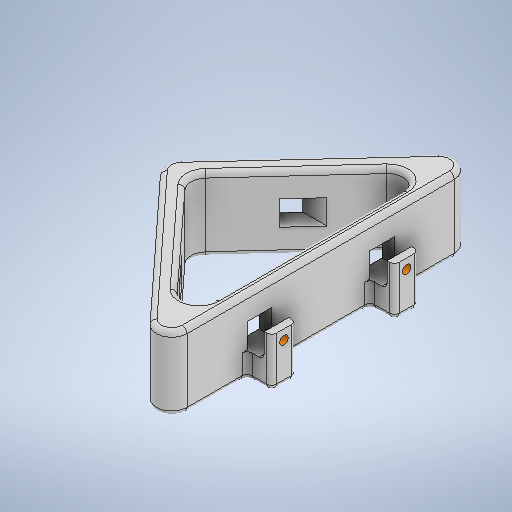
# Autodesk Inventor part: pare-chocs
Saved by Autodesk Inventor 2025 (Build 290162000, 162)
## iProperties
Created: 2024-10-10
Part Number: pare-chocs
Material: Générique
Document SubType Name: Modeling
Designer: chass
Density: 1 g/cm^3
Appearance: Par défaut
Author: chass
## iProperties of the stored document pare-chocs_Impression 3D.ipt
Created: 2025-01-09
Part Number: pare-chocs_Impression 3D
Material: Générique
Document SubType Name: Modeling
Designer: chass
Density: 1 g/cm^3
Appearance: Par défaut
Author: chass
Autodesk Inventor part; units mm, degrees
ref_plane "YZ Plane" through (0, 0, 0) normal (1, 0, 0) x (0, 1, 0)
ref_plane "XZ Plane" through (0, 0, 0) normal (0, 1, 0) x (-1, 0, 0)
ref_plane "XY Plane" through (0, 0, 0) normal (0, 0, 1) x (1, 0, 0)
sketch "Esquisse1" plane through (0, 0, 0) normal (1, 0, 0) x (0, 1, 0)
  line L0 (-2.5, 65) -> (2.5, 65)
  line L1 (2.5, 65) -> (2.5, -65)
  line L2 (2.5, -65) -> (-2.5, -65)
  line L3 (-2.5, -65) -> (-2.5, 65)
  line L4 (2.5, 65) -> (-2.5, -65)
  line L5 (2.5, -65) -> (-2.5, 65)
  point P0 (0, 0)
  point P1 (0, 0)
  point P2 (0, 0)
  dimension "d0" = 130
  dimension "d1" = 5
  constraints: 12 end point, 2 midpoint, 2 parallel, 1 coincident, 1 horizontal, 1 perpendicular
  measures "d0" distance of L0.end L1.end
  measures "d1" distance of L1.end L2.end
extrude "Extrusion1" add sketch "Esquisse1" along normal blind 5
sketch "Esquisse2" plane through (5, 0, 0) normal (1, 0, 0) x (0, 0, -1)
  line L0 (65, 2.5) -> (-65, 2.5) projected
  line L1 (-65, -2.5) -> (65, -2.5) projected
  line L2 (-30, 2.5) -> (-20, 2.5)
  line L3 (-20, 2.5) -> (-20, -2.5)
  line L4 (-20, -2.5) -> (-30, -2.5)
  line L5 (-30, -2.5) -> (-30, 2.5)
  line L6 (0, 13) -> (0, -16)
  line L7 (30, 2.5) -> (20, 2.5)
  line L8 (20, 2.5) -> (20, -2.5)
  line L9 (20, -2.5) -> (30, -2.5)
  line L10 (30, -2.5) -> (30, 2.5)
  point P0 (0, 0)
  point P1 (-20, 2.5)
  point P2 (30, -2.5)
  point P3 (30, 2.5)
  point P4 (20, 2.5)
  point P5 (20, -2.5)
  dimension "d4" = 10
  dimension "d5" = 20
  constraints: 18 end point, 4 symmetric about line, 3 point on line, 2 parallel, 1 horizontal, 1 perpendicular, 1 vertical
  measures "d4" distance between parallel lines of L3 L5
  measures "d5" distance between parallel lines of L3 L6
extrude "Extrusion2" add sketch "Esquisse2" along normal blind 10 contours L10 L1 L8 L0 | L3 L1 L5 L0
sketch "Esquisse3" plane through (0, 2.5, 65) normal (0, 1, 0) x (1, 0, 0)
  line L0 (15, 45) -> (15, 35) projected
  line L1 (5, 45) -> (15, 45) projected
  line L2 (15, 35) -> (12, 35)
  line L3 (12, 35) -> (12, 45)
  line L4 (12, 45) -> (15, 45)
  line L5 (15, 45) -> (15, 35)
  line L6 (-9, 65) -> (24, 65)
  line L7 (15, 85) -> (15, 95)
  line L8 (15, 95) -> (12, 95)
  line L9 (12, 95) -> (12, 85)
  line L10 (12, 85) -> (15, 85)
  line L11 (15, 85) -> (15, 95)
  point P0 (0, 65)
  constraints: 20 end point, 5 symmetric about line, 2 horizontal, 2 parallel, 1 perpendicular, 1 point on line
extrude "Extrusion3" add sketch "Esquisse3" along normal blind 15
sketch "Esquisse4" plane through (15, 0, 0) normal (1, 0, 0) x (0, 0, -1)
  circle A0 centre (-25, 13.5) radius 1.75
  line L0 (0, 20) -> (0, -21)
  circle A1 centre (25, 13.5) radius 1.75
  line L1 (-30, 17.5) -> (-20, 17.5) projected
  line L2 (-20, -2.5) -> (-20, 17.5) projected
  point P0 (0, 0)
  dimension "d10" = 3.5
  dimension "d11" = 4
  dimension "d19" = 5
  constraints: 2 centre point, 2 end point, 1 symmetric about line, 1 vertical, 1 other
  measures "d10" diameter of A0
  measures "d11" distance from line of L1 A0.centre
  measures "d19" distance from line of L2 A0.centre
extrude "Extrusion4" cut sketch "Esquisse4" against normal blind 10
sketch "Esquisse12" plane through (0, -2.5, -65) normal (0, -1, 0) x (1, 0, 0)
  line L0 (0, 130) -> (0, 0) projected
  line L1 (0, 0) -> (5, 0) projected
  line L2 (0, 0) -> (5, 0)
  line L3 (5, 0) -> (5, 130)
  line L4 (5, 130) -> (0, 130)
  line L5 (0, 130) -> (-60, 65)
  line L6 (-60, 65) -> (0, 0)
  line L7 (0, 0) -> (0, 130) projected
  line L8 (0, 130) -> (5, 130) projected
  point P0 (0, 65)
  point P1 (0, 65)
  dimension "d41" = 60
  constraints: 10 end point, 2 perpendicular, 1 collinear, 1 horizontal, 1 midpoint
  measures "d41" distance of L5.end point (0, 65)
extrude "Extrusion9" add sketch "Esquisse12" against normal blind 30
sketch "Esquisse13" plane through (5, 2.5, -20) normal (0, 1, 0) x (1, 0, 0)
  line L0 (0, 0) -> (7, 0) projected
  line L1 (7, 0) -> (0, 0)
  line L2 (0, 0) -> (0, 10)
  line L3 (0, 10) -> (7, 10)
  line L4 (7, 10) -> (7, 0)
  line L5 (7, -50) -> (0, -50)
  line L6 (0, -50) -> (0, -40)
  line L7 (0, -40) -> (7, -40)
  line L8 (7, -40) -> (7, -50)
  point P0 (-5, -20)
  constraints: 16 end point, 4 parallel, 2 horizontal, 2 perpendicular, 2 point on line
extrude "Extrusion10" add sketch "Esquisse13" along normal blind 7
sketch "Esquisse14" plane through (0, 27.5, -65) normal (0, 1, 0) x (1, 0, 0)
  line L0 (0, -18.125) -> (0, -111.875)
  line L1 (0, -111.875) -> (-7, -111.875)
  line L2 (-7, -111.875) -> (-50, -65)
  line L3 (-50, -65) -> (-7, -18.125)
  line L4 (-7, -18.125) -> (0, -18.125)
  point P0 (0, -65)
  point P1 (0, -65)
  dimension "d42" = 50
  dimension "d43" = 0
  dimension "d44" = 7
  constraints: 10 end point, 2 parallel, 1 midpoint, 1 perpendicular, 1 vertical
  measures "d42" distance of L2.end point (0, -65)
  measures "d43" distance from line of L0 point (0, -65)
  measures "d44" distance of L0.end L1.end
extrude "Extrusion11" cut sketch "Esquisse14" against normal blind 44
sketch "Esquisse16" plane through (12, 17.5, -30) normal (-1, 0, 0) x (0, 0, 1)
  line L0 (0, -20) -> (0, 0) projected
  line L1 (10, -20) -> (10, 0) projected
  line L2 (0, 0) -> (10, 0)
  line L3 (10, 0) -> (10, -10)
  line L4 (10, -10) -> (0, -10)
  line L5 (0, -10) -> (0, 0)
  line L6 (50, -20) -> (50, 0) projected
  line L7 (60, -20) -> (60, 0) projected
  line L8 (50, 0) -> (60, 0)
  line L9 (60, 0) -> (60, -10)
  line L10 (60, -10) -> (50, -10)
  line L11 (50, -10) -> (50, 0)
  point P0 (30, -17.5)
  point P1 (50, -10)
  point P2 (0, -10)
  constraints: 16 end point, 4 parallel, 2 horizontal, 2 midpoint, 2 perpendicular
extrude "Extrusion13" cut sketch "Esquisse16" along normal blind 79.75
fillet "Congé15" radius 6.25 1 edges at (-60, 12.5, 0)
fillet "Congé16" radius 6.25 5 edges at (-7, 12.5, -46.875) (0, 12.5, -46.875) (-50, 12.5, 0) (-7, 12.5, 46.875) (0, 12.5, 46.875)
fillet "Congé17" radius 6.25 4 edges at (5, 12.5, 65) (0, 12.5, 65) (5, 12.5, -65) (0, 12.5, -65)
fillet "Congé18" radius 2 8 edges at (12, 7.5, -25) (12, 7.5, 25) (15, -2.5, -25) (15, -2.5, 25) (5, 2.5, 30) (5, 2.5, 20) (5, 2.5, -20) (5, 2.5, -30)
fillet "Congé19" radius 2 29 edges at (-30.9638, -2.5, 31.4559) (-57.7443, -2.5, 0) (-30.9638, -2.5, -31.4559) (5, -2.5, -43.217) (5.5858, -2.5, -30.5858) (10, -2.5, -30) (14.4142, -1.9142, -30) (15, 8.5, -30) (5, -2.5, 43.217) (5.5858, -2.5, 30.5858) (10, -2.5, 30) (14.4142, -1.9142, 30) (15, 8.5, 30) (5, 27.5, 0) (-30.9638, 27.5, -31.4559) (-57.7443, 27.5, 0) (-30.9638, 27.5, 31.4559) (-3.9825, 27.5, -44.273) (0, 27.5, 0) (-3.9825, 27.5, 44.273) (-28.4891, 27.5, 23.4493) (-47.7686, 27.5, 0) (-28.4891, 27.5, -23.4493) (-3.9825, -2.5, 44.273) (0, -2.5, 0) (-3.9825, -2.5, -44.273) (-28.4891, -2.5, -23.4493) (-47.7686, -2.5, 0) (-28.4891, -2.5, 23.4493)
fillet "Congé20" radius 2 9 edges at (14.4142, -1.9142, 20) (10, -2.5, 20) (5.5858, -2.5, 19.4142) (5, -2.5, 0) (5.5858, -2.5, -19.4142) (10, -2.5, -20) (14.4142, -1.9142, -20) (15, 8.5, -20) (15, 8.5, 20)
